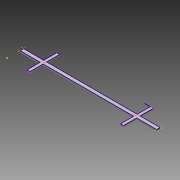
# Autodesk Inventor part: Brace
Saved by Autodesk Inventor 2015 (Build 190159000, 159)
## iProperties
Created: 2016-01-15
Part Number: Brace
Material: ABS Plastic
Document SubType Name: Modeling
Designer: 576994
Mass: 64.2385 g
Surface Area: 282.063 cm^2
Volume: 60.6023 cm^3
Density: 1.06 g/cm^3
Appearance: Smooth - White
Author: 576994
Autodesk Inventor part; units mm, degrees
ref_plane "Work Plane4" through (0, 0, 5) normal (0, 0, 1) x (1, 0, 0)
sketch "Sketch2" plane through (0, 0, 5) normal (0, 0, 1) x (1, 0, 0)
  line L0 (0, 0) -> (235, 0)
  line L1 (235, 0) -> (235, 51)
  line L2 (235, 51) -> (0, 51)
  line L3 (0, 51) -> (0, 0)
  line L4 (235, 0) -> (235, 51) projected
  line L5 (0, 22.5) -> (235, 22.5)
  line L6 (235, 22.5) -> (235, 28.5)
  line L7 (235, 28.5) -> (0, 28.5)
  line L8 (0, 28.5) -> (0, 22.5)
  line L9 (0, 22.5) -> (235, 28.5) construction
  line L10 (235, 22.5) -> (0, 28.5) construction
  point P0 (117.5, 25.5)
  dimension "d4" = 6
  constraints: 20 end point, 4 parallel, 2 horizontal, 2 midpoint, 2 perpendicular, 1 point on line
  measures "d4" distance of L6.end L5.end
extrude "Extrusion2" add sketch "Sketch2" along normal blind 3 contours L3 L7 L1 L5
ref_plane "Work Plane8" through (0, 0, 5) normal (0, 0, 1) x (1, 0, 0)
sketch "Sketch3" plane through (0, 0, 5) normal (0, 0, 1) x (1, 0, 0)
  line L0 (0, 28.5) -> (235, 28.5) projected
  line L1 (235, 51) -> (0, 51) projected
  line L2 (34.5, 28.5) -> (39.5, 28.5)
  line L3 (39.5, 28.5) -> (39.5, 51)
  line L4 (39.5, 51) -> (34.5, 51)
  line L5 (34.5, 51) -> (34.5, 28.5)
  point P0 (0, 0)
  dimension "d7" = 5
  constraints: 8 end point, 2 parallel, 2 point on line, 1 horizontal, 1 perpendicular
  measures "d7" distance of L4.end L3.end
ref_plane "Work Plane9" through (0, 0, 5) normal (0, 0, 1) x (1, 0, 0)
sketch "Sketch5" plane through (0, 0, 5) normal (0, 0, 1) x (1, 0, 0)
  line L0 (235, 51) -> (0, 51) projected
  line L1 (117.5, 51) -> (117.5, 0)
  line L2 (235, 28.5) -> (0, 28.5) projected
  line L3 (34.5, 51) -> (39.5, 51)
  line L4 (39.5, 51) -> (39.5, 28.5)
  line L5 (39.5, 28.5) -> (34.5, 28.5)
  line L6 (34.5, 28.5) -> (34.5, 51)
  line L7 (0, 22.5) -> (235, 22.5) projected
  line L8 (34.5, 22.5) -> (39.5, 22.5)
  line L9 (39.5, 22.5) -> (39.5, 0)
  line L10 (39.5, 0) -> (34.5, 0)
  line L11 (34.5, 0) -> (34.5, 22.5)
  line L12 (195.5, 51) -> (195.5, 28.5)
  line L13 (200.5, 28.5) -> (200.5, 51)
  line L14 (195.5, 22.5) -> (195.5, 0)
  line L15 (195.5, 0) -> (200.5, 0)
  line L16 (200.5, 0) -> (200.5, 22.5)
  line L17 (195.5, 28.5) -> (200.5, 28.5)
  line L18 (195.5, 22.5) -> (200.5, 22.5)
  line L19 (195.5, 51) -> (200.5, 51)
  point P0 (0, 0)
  dimension "d13" = 5
  constraints: 34 end point, 8 symmetric about line, 4 parallel, 3 perpendicular, 3 point on line, 2 collinear, 2 horizontal, 1 midpoint, 1 vertical
  measures "d13" distance of L4.end L5.end
extrude "Extrusion5" add sketch "Sketch3" along normal blind 3
extrude "Extrusion6" add sketch "Sketch5" along normal blind 3 contours L9 L10 L11 L7
extrude "Extrusion7" add sketch "Sketch5" along normal blind 3 contours L13 L2 L12 L0 | L7 L16 L15 L14
sketch "Sketch7" plane through (0, 0, 8) normal (0, 0, 1) x (1, 0, 0)
  line L0 (0, 28.5) -> (34.5, 28.5)
  line L1 (34.5, 28.5) -> (34.5, 51)
  line L2 (34.5, 51) -> (39.5, 51)
  line L3 (39.5, 51) -> (39.5, 28.5)
  line L4 (39.5, 28.5) -> (39.5, 51) projected
  line L5 (39.5, 28.5) -> (195.5, 28.5)
  line L6 (195.5, 28.5) -> (195.5, 51)
  line L7 (195.5, 51) -> (195.5, 28.5) projected
  line L8 (195.5, 51) -> (185.7081, 51)
  line L9 (200.5, 51) -> (200.5, 28.5)
  line L10 (200.5, 28.5) -> (200.5, 51) projected
  line L11 (200.5, 28.5) -> (235, 28.5)
  line L12 (235, 28.5) -> (235, 22.5)
  line L13 (235, 22.5) -> (200.5, 22.5)
  line L14 (200.5, 22.5) -> (200.5, 0)
  line L15 (200.5, 0) -> (200.5, 22.5) projected
  line L16 (200.5, 0) -> (195.5, 0)
  line L17 (195.5, 0) -> (200.5, 0) projected
  line L18 (195.5, 0) -> (195.5, 22.5)
  line L19 (195.5, 22.5) -> (39.5, 22.5)
  line L20 (0, 22.5) -> (235, 22.5) projected
  line L21 (39.5, 22.5) -> (39.5, 0)
  line L22 (39.5, 0) -> (34.5, 0)
  line L23 (34.5, 0) -> (39.5, 0) projected
  line L24 (34.5, 0) -> (34.5, 22.5)
  line L25 (34.5, 22.5) -> (34.5, 0) projected
  line L26 (34.5, 22.5) -> (0, 22.5)
  line L27 (0, 22.5) -> (0, 28.5)
  line L28 (0, 28.5) -> (0, 22.5) projected
  point P0 (0, 0)
  constraints: 40 end point, 9 collinear, 9 perpendicular, 2 point on line, 1 horizontal
body "Solid1"
